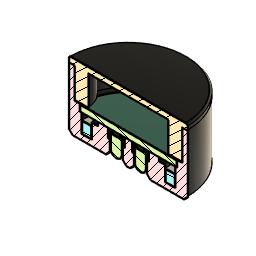
smartmeter-reading-head (Autodesk Fusion 360 design; units mm, degrees)
Autodesk Fusion 360 part; units mm, degrees
note: some values were not read from the file. Chosen so that the rebuilt part matches the saved one: which face or edge a step refers to. Set by a fixed rule: which sketch regions a step uses.
sketch "Sketch1" plane through (0, 0, 0) normal (0, 0, 1) x (1, 0, 0) in component "Gehäuse"
  circle A0 centre (0, 0) radius 16
  circle A1 centre (0, 0) radius 12.625
  circle A2 centre (0, 0) radius 9.875
  circle A3 centre (-3.25, 0) radius 1.75
  circle A4 centre (3.25, 0) radius 1.75
  line L0 (0, 18) -> (0, -18) construction
  line L1 (-18, 0) -> (18, 0) construction
  circle A5 centre (0, 0) radius 13.125
  circle A6 centre (-3.25, 0) radius 2.25
  circle A7 centre (3.25, 0) radius 2.25
  line L2 (-3.25, 5) -> (3.25, 5)
  line L3 (-3.25, -5) -> (3.25, -5)
  arc A8 (-3.25, 5) -> (-3.25, -5) centre (-3.25, 0) ccw
  arc A9 (3.25, -5) -> (3.25, 5) centre (3.25, 0) ccw
  dimension "d1" = 32
  dimension "d2" = 25.25
  dimension "d3" = 19.75
  dimension "d4" = 3.5
  dimension "d5" = 6.5
  dimension "d20" = 26.25
  dimension "d29" = 4.5
  dimension "d91" = 10
  constraint coincident A0.centre A1.centre
  constraint concentric A1 A2
  constraint equal A3 A4
  constraint vertical L0
  constraint perpendicular L0 L1
  constraint coincident A3.centre L1
  constraint coincident A4.centre L1
  constraint symmetric A3 A4 L0
  constraint midpoint A0.centre L0
  constraint midpoint A0.centre L1
  constraint concentric A0 A5
  constraint concentric A3 A6
  constraint symmetric L0 A6 A7
  constraint concentric A3 A8
  constraint perpendicular L0 L2
  constraint perpendicular L0 L3
  constraint tangent L2 A8
  constraint tangent L3 A8
  constraint symmetric L0 L2.start L2.end
  constraint symmetric L0 L3.start L3.end
  constraint symmetric L0 A8 A9
  measures "d1" diameter of A0
  measures "d2" diameter of A1
  measures "d3" diameter of A2
  measures "d4" diameter of A3
  measures "d5" distance of A3.centre A4.centre
  measures "d20" diameter of A5
  measures "d29" diameter of A6
  measures "d91" diameter of A8
extrude "Extrude1" add sketch "Sketch1" along normal blind 16.5 contours A0 | A1 | A2 | A3 | A4 | A5 | A6 | A7 | L2 L3 A8 A9 makes body 1 in component "Gehäuse"
shell "Shell1" thickness 1.5 removed faces 1 at (3.3126, -0.5422, 16.5) on bodies 1 in component "Gehäuse"
extrude "Extrude3" add sketch "Sketch1" along normal blind 5 from surface at 1.5 contours A0 | A2 | A3 | A4 | A5 | A6 | A7 | L2 L3 A8 A9 bodies 1 in component "Gehäuse"
extrude "Extrude4" add sketch "Sketch1" along normal blind 1.8 from surface at 6.5 contours A0 bodies 1 in component "Gehäuse"
extrude "Extrude6" cut sketch "Sketch1" against normal blind 1 from surface at 6.5 contours A2 bodies 1 in component "Gehäuse"
extrude "Extrude2" cut sketch "Sketch1" along normal through all contours A3 | A4 bodies 1 in component "Gehäuse"
extrude "Extrude5" cut sketch "Sketch1" along normal up to surface (2.5 mm away) from surface at 4 contours A3 | A4 | A6 | A7 bodies 1 in component "Gehäuse"
chamfer "Chamfer1" distance 1 angle 45 1 edges at (-14.9172, -5.7858, 0) on bodies 1 in component "Gehäuse"
chamfer "Chamfer1" distance 1 angle 45 2 edges at (-4.8816, -0.6328, 0) (1.6184, -0.6328, 0) on bodies 1 in component "Gehäuse"
hole "Hole1" at (0, -16, 10.6688) direction (0, 1, 0) diameter 4 depth 2 tip angle 180 bodies 1 in component "Gehäuse"
sketch "Sketch1 (2)" plane through (0, 0, 1.5) normal (0, 0, 1) x (-1, 0, 0) in component "Magnet"
  circle A0 centre (3.25, 0) radius 1.75
  circle A1 centre (-3.25, 0) radius 1.75
  circle A2 centre (0, 0) radius 9.875
  circle A3 centre (0, 0) radius 12.5
  circle A4 centre (0, 0) radius 10
  circle A5 centre (0, 0) radius 9.875
  circle A6 centre (0, 0) radius 12.625
  dimension "d12" = 25
  dimension "d13" = 20
  constraint coincident A2.centre A3.centre
  measures "d12" diameter of A3
  measures "d13" diameter of A4
extrude "Extrude1'" add sketch "Sketch1 (2)" along normal blind 3 from surface at 0.1 separate body contours A3 makes body 2 in component "Magnet"
sketch "Sketch1 (3)" plane through (0, 0, 6.5) normal (0, 0, 1) x (1, 0, 0) in component "PCB"
  circle A0 centre (0, 0) radius 13
  line L0 (0, 15) -> (0, -15) construction
  line L1 (-15, 0) -> (15, 0) construction
  circle A1 centre (-3.25, 0) radius 1.5
  circle A2 centre (3.25, 0) radius 1.5
  circle A3 centre (-3.25, 0) radius 2
  circle A4 centre (3.25, 0) radius 2
  circle A5 centre (-4.52, 0) radius 0.25
  line L2 (-3.25, -1) -> (-3.25, 1) construction
  circle A6 centre (-1.98, 0) radius 0.25
  circle A7 centre (4.52, 0) radius 0.25
  circle A8 centre (1.98, 0) radius 0.25
  circle A9 centre (0, 0) radius 12.625
  circle A10 centre (0, 0) radius 13.125
  dimension "d21" = 26
  dimension "d32" = 3
  dimension "d33" = 6.5
  dimension "d34" = 4
  dimension "d46" = 0.5
  dimension "d47" = 2.54
  constraint coincident A0.centre A9.centre
  constraint vertical L0
  constraint midpoint A0.centre L0
  constraint horizontal L1
  constraint midpoint A0.centre L1
  constraint coincident L1 A1.centre
  constraint symmetric L0 A1 A2
  constraint concentric A1 A3
  constraint symmetric L0 A3 A4
  constraint coincident L1 A5.centre
  constraint vertical L2
  constraint midpoint A1.centre L2
  constraint symmetric A5 L2 A6
  constraint symmetric L0 A5 A7
  constraint symmetric L0 A6 A8
  measures "d21" diameter of A0
  measures "d32" diameter of A1
  measures "d33" distance of A1.centre A2.centre
  measures "d34" diameter of A3
  measures "d46" diameter of A5
  measures "d47" distance of A5.centre A6.centre
extrude "Extrude1''" add sketch "Sketch1 (3)" along normal blind 1.6 separate body contours A0 | A1 A6 | A1 A6 | A1 A5 A6 | A1 A5 | A1 A5 | A2 A7 | A2 A7 | A2 A7 A8 | A2 A8 | A2 A8 | A3 | A4 | A9 makes body 3 in component "PCB"
extrude "Extrude5'" add sketch "Sketch1 (3)" against normal blind 1 separate body contours A1 A6 | A1 A5 | A2 A7 | A2 A8 picked at (-2.0696, 0) picked at (-4.5897, 0) picked at (4.4304, 0) picked at (1.9103, 0) makes body 4 at (-1.7652, -0.1279, 6.1667) makes body 5 at (2.0136, -0.2477, 6.1667) makes body 6 at (-4.5947, 0.2386, 5.8333) makes body 7 at (4.7348, -0.1279, 5.8333) in component "PCB"
extrude "Extrude6'" add sketch "Sketch1 (3)" against normal blind 1 from surface at -1 contours A1 A6 | A1 A5 A6 | A1 A5 | A2 A7 | A2 A7 A8 | A2 A8 | A3 | A4 picked at (-2.0696, 0) picked at (-4.5897, 0) picked at (4.4304, 0) picked at (1.9103, 0) bodies 4 5 6 7 in component "PCB"
extrude "Extrude7" add sketch "Sketch1 (3)" against normal blind 4 from surface at -2 contours A1 A6 | A1 A5 A6 | A1 A5 | A2 A7 | A2 A7 A8 | A2 A8 picked at (-2.0696, 0) picked at (-4.5897, 0) picked at (4.4304, 0) picked at (1.9103, 0) bodies 4 5 in component "PCB"
fillet "Fillet2" radius 1.5 2 edges at (-4.6485, 0.5424, 0.5) (1.8515, 0.5424, 0.5) on bodies 4 5 in component "PCB"
sketch "Sketch1 (4)" plane through (0, 0, 16.5) normal (0, 0, 1) x (1, 0, 0) in component "Deckel"
  circle A0 centre (0, 0) radius 16
  circle A1 centre (0, 0) radius 14.5
  circle A2 centre (0, 0) radius 13
  circle A3 centre (0, 0) radius 14.5
  circle A4 centre (0, 0) radius 16
  line L0 (-20, 0) -> (20, 0) construction
  arc A5 (-13.6107, -5) -> (-13.6107, 5) centre (-16.5, 0) ccw
  line L1 (0, 20) -> (0, -20) construction
  arc A6 (13.6107, 5) -> (13.6107, -5) centre (16.5, 0) ccw
  dimension "d75" = 32
  dimension "d76" = 29
  dimension "d79" = 26
  dimension "d96" = 10
  dimension "d97" = 33
  constraint coincident A0.centre A1.centre
  constraint concentric A0 A1
  constraint concentric A0 A2
  constraint horizontal L0
  constraint midpoint A0.centre L0
  constraint coincident A3 A5.start
  constraint coincident A3 A5.end
  constraint coincident L0 A5.centre
  constraint vertical L1
  constraint midpoint A0.centre L1
  constraint symmetric A5.end L1 A6.start
  constraint symmetric A5.start L1 A6.end
  constraint symmetric A5 L1 A6
  measures "d75" diameter of A0
  measures "d76" diameter of A1
  measures "d79" diameter of A2
  measures "d96" vertical distance of A5.end A5.start
  measures "d97" distance of A5.centre A6.centre
extrude "Extrude3'" add sketch "Sketch1 (4)" along normal blind 1.5 separate body contours A0 A4 | A1 A2 A3 A6 | A1 A2 A3 A5 A6 | A1 A2 A3 A5 A6 | A1 A2 A3 A5 | A2 A5 A6 | A2 A6 | A2 A5 makes body 8 in component "Deckel"
extrude "Extrude4'" add sketch "Sketch1 (4)" against normal blind 3 contours A1 A2 A3 A6 | A1 A2 A3 A5 A6 | A1 A2 A3 A5 A6 | A1 A2 A3 A5 bodies 8 in component "Deckel"
extrude "Extrude5''" add sketch "Sketch1 (4)" against normal blind 8 contours A1 A2 A3 A6 | A1 A2 A3 A5 | A2 A6 | A2 A5 bodies 8 in component "Deckel"
fillet "Fillet1" radius 0.5 1 edges at (-14.9172, -5.7858, 18) on bodies 8 in component "Deckel"
chamfer "Chamfer1'" distance 0.25 angle 45 2 edges at (0, 14.5, 13.5) (0, -14.5, 13.5) on bodies 8 in component "Deckel"
component "Gehäuse" placed x (1, 0, 0) y (0, 1, 0) z (0, 0, 1) at (0, 0, 0)
component "Deckel" placed x (1, 0, 0) y (0, 1, 0) z (0, 0, 1) at (0, 0, 0)
component "Magnet" placed x (1, 0, 0) y (0, 1, 0) z (0, 0, 1) at (0, 0, 0)
component "PCB" placed x (1, 0, 0) y (0, 1, 0) z (0, 0, 1) at (0, 0, 0)
equation "d2 = 25 mm + 0.25 mm"
equation "d3 = 20 mm - 0.25 mm"
equation "d4 = 3 mm + 0.5 mm"
equation "d20 = 26 mm + 0.25 mm"
named bodies: "Gehäuse", "Magnet", "PCB", "LED1", "LED2", "Deckel"
